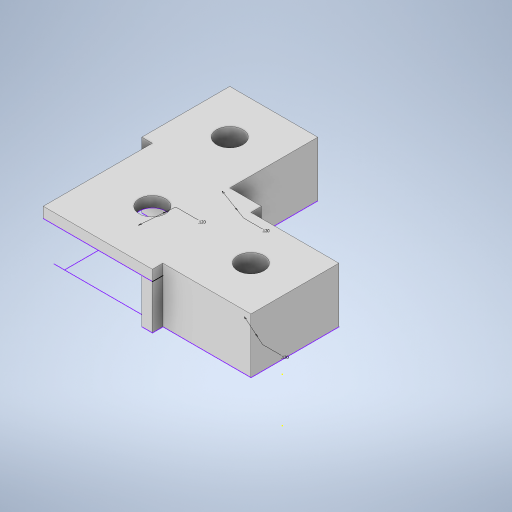
# Autodesk Inventor part: tab
Saved by Autodesk Inventor 2024 (Build 280153000, 153)
## iProperties
Created: 2023-04-14
Part Number: tab
Material: Generic
Document SubType Name: Modeling
Designer: Fujitsu
Density: 1 g/cm^3
Appearance: Default
Author: Fujitsu
Autodesk Inventor part; units mm, degrees
ref_plane "YZ Plane" through (0, 0, 0) normal (1, 0, 0) x (0, 1, 0)
ref_plane "XZ Plane" through (0, 0, 0) normal (0, 1, 0) x (-1, 0, 0)
ref_plane "XY Plane" through (0, 0, 0) normal (0, 0, 1) x (1, 0, 0)
sketch "Sketch1" plane through (0, 0, 0) normal (0, 1, 0) x (-1, 0, 0)
  line L0 (16.7831, -1.7829) -> (16.7831, -14.3813)
  line L1 (16.7831, -14.3813) -> (29.3815, -14.3813)
  line L2 (28.1623, -3.0021) -> (18.0023, -3.0021)
  line L3 (18.0023, -3.0021) -> (18.0023, -13.1621)
  line L4 (18.0023, -13.1621) -> (28.1623, -13.1621)
  line L5 (28.1623, -13.1621) -> (28.1623, -3.0021)
  line L6 (28.1623, -3.0021) -> (29.3815, -3.0021)
  line L7 (30.6007, -14.3813) -> (20.4407, -14.3813)
  line L8 (20.4407, -14.3813) -> (20.4407, -24.5413)
  line L9 (20.4407, -24.5413) -> (30.6007, -24.5413)
  line L10 (30.6007, -24.5413) -> (30.6007, -14.3813)
  line L11 (16.7831, -3.0021) -> (6.6231, -3.0021)
  line L12 (6.6231, -3.0021) -> (6.6231, -13.1621)
  line L13 (6.6231, -13.1621) -> (16.7831, -13.1621)
  line L14 (16.7831, -13.1621) -> (16.7831, -3.0021)
  line L15 (28.1623, -13.1621) -> (29.3815, -13.1621)
  line L16 (18.0023, -3.0021) -> (18.0023, -1.7829)
  line L17 (29.3815, -13.1621) -> (29.3815, -14.3813)
  line L18 (18.0023, -1.7829) -> (16.7831, -1.7829)
  line L19 (18.0023, -1.7829) -> (16.7831, -1.7829)
  circle A0 centre (25.5207, -19.4613) radius 1.524
  circle A1 centre (11.7031, -8.0821) radius 1.524
  point P0 (0, 0)
  dimension "d16" = 3.048
  dimension "d17" = 3.048
  constraints: 40 end point, 4 point on line, 2 centre point
  measures "d16" diameter of A0
  measures "d17" diameter of A1
extrude "Extrusion1" add sketch "Sketch1" along normal blind 5.1308 contours L18 L16 L3 L4 L15 L17 L1 L0
sketch "Sketch2" plane through (0, 5.1308, 0) normal (0, 1, 0) x (1, 0, 0)
  line L0 (-16.7831, 14.3813) -> (-29.3815, 14.3813) projected
  line L1 (-16.7831, 14.3813) -> (-29.3815, 14.3813)
  line L2 (-29.3815, 14.3813) -> (-29.3815, 1.7884)
  line L3 (-29.3815, 1.7884) -> (-16.7831, 1.7884)
  line L4 (-16.7831, 1.7884) -> (-16.7831, 14.3813)
  circle A0 centre (-23.0823, 8.0848) radius 1.524
  point P0 (0, 0)
  dimension "d4" = 3.048
  constraints: 8 end point, 2 parallel, 1 centre point, 1 horizontal, 1 perpendicular
  measures "d4" diameter of A0
extrude "Extrusion2" add sketch "Sketch2" along normal blind 1.2192 contours L4 L3 L2 L0 | A0
hole "Hole1" at (-23.0823, 5.1308, -8.0848) direction (0, 1, 0) diameter 3.048 end through all
extrude "Extrusion3" add sketch "Sketch1" along normal blind 6.35 contours L1 L7 L10 L9 L8 | A0
extrude "Extrusion4" add sketch "Sketch1" along normal blind 6.35 contours L0 L13 L12 L11 | A1
hole "Hole2" at (-11.7031, 0, -8.0821) direction (0, 1, 0) diameter 3.048 end through all
hole "Hole3" at (-25.5207, 0, -19.4613) direction (0, 1, 0) diameter 3.048 end through all
body "Solid1"
